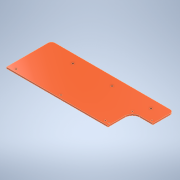
# Autodesk Inventor part: Electronics cover
Saved by Autodesk Inventor 2021 (Build 250183000, 183)
## iProperties
Created: 2020-08-17
Part Number: Electronics cover
Material: Generic
Document SubType Name: Modeling
Designer: jgray
Density: 1 g/cm^3
Appearance: Smooth - Light Orange
Author: jgray
Autodesk Inventor part; units mm, degrees
ref_plane "YZ Plane" through (0, 0, 0) normal (1, 0, 0) x (0, 1, 0)
ref_plane "XZ Plane" through (0, 0, 0) normal (0, 1, 0) x (-1, 0, 0)
ref_plane "XY Plane" through (0, 0, 0) normal (0, 0, 1) x (1, 0, 0)
sketch "Sketch1" plane through (0, 0, 0) normal (0, 1, 0) x (-1, 0, 0)
  line L0 (0, 0) -> (250, 0)
  line L1 (250, 0) -> (250, -85.25)
  line L2 (243, -92.25) -> (7, -92.25)
  line L3 (0, -85.25) -> (0, 0)
  arc A0 (243, -92.25) -> (250, -85.25) centre (243, -85.25) ccw
  arc A1 (0, -85.25) -> (7, -92.25) centre (7, -85.25) ccw
  point P0 (250, -92.25)
  point P1 (0, -92.25)
  dimension "d0" = 250
  dimension "d1" = 92.25
  dimension "d2" = 7
  constraints: 8 end point, 4 point on circle, 4 point on line, 4 tangent, 2 centre point, 2 parallel, 1 equal radius, 1 horizontal, 1 perpendicular
  measures "d0" distance of point (250, -92.25) point (0, -92.25)
  measures "d1" distance of L0.end point (250, -92.25)
  measures "d2" radius of A0
extrude "Extrusion1" add sketch "Sketch1" along normal blind 3
sketch "Sketch2" plane through (0, 3, 0) normal (0, 1, 0) x (1, 0, 0)
  line L0 (-302.172, 6) -> (59.9962, 6) construction
  line L1 (-309.1368, 74) -> (37.3606, 74) construction
  line L2 (-7, 92.25) -> (-243, 92.25) projected
  line L3 (-250, 0) -> (0, 0) projected
  line L4 (0, 0) -> (0, 85.25) projected
  line L5 (-250, 85.25) -> (-250, 0) projected
  point P0 (-28, 74)
  point P1 (-108, 74)
  point P2 (-188, 74)
  point P3 (-53.5, 6)
  point P4 (-144.5, 6)
  point P5 (-236.5, 6)
  dimension "d5" = 18.25
  dimension "d6" = 6
  dimension "d8" = 80
  dimension "d9" = 80
  dimension "d20" = 13.5
  dimension "d22" = 196.5
  dimension "d23" = 62
  dimension "d24" = 105.5
  constraints: 6 point on line, 4 end point, 2 horizontal
  measures "d5" distance between parallel lines of L2 L1
  measures "d6" distance between parallel lines of L3 L0
  measures "d8" distance of point (-28, 74) point (-108, 74)
  measures "d9" distance of point (-108, 74) point (-188, 74)
  measures "d20" distance from line of L5 point (-236.5, 6)
  measures "d22" distance from line of L5 point (-53.5, 6)
  measures "d23" distance from line of L5 point (-188, 74)
  measures "d24" distance from line of L5 point (-144.5, 6)
hole "Hole1" at (-28, 3, -74) at (-108, 3, -74) at (-188, 3, -74) at (-53.5, 3, -6) at (-144.5, 3, -6) at (-236.5, 3, -6) direction (0, -1, 0) diameter 3.8 end through all
sketch "Sketch3" plane through (0, 3, 0) normal (0, 1, 0) x (1, 0, 0)
  line L0 (0, 0) -> (-42, 0)
  line L1 (-42, 0) -> (-42, 35)
  line L2 (-27, 50) -> (0, 50)
  line L3 (0, 50) -> (0, 0)
  line L4 (-250, 85.25) -> (-250, 0) projected
  arc A0 (-27, 50) -> (-42, 35) centre (-27, 35) ccw
  dimension "d26" = 50
  dimension "d27" = 208
  dimension "d28" = 15
  constraints: 8 end point, 2 parallel, 2 point on circle, 2 tangent, 1 centre point, 1 horizontal, 1 perpendicular
  measures "d26" distance between parallel lines of L0 L2
  measures "d27" distance between parallel lines of L4 L1
  measures "d28" radius of A0
extrude "Extrusion2" cut sketch "Sketch3" against normal through all
sketch "Sketch4" plane through (0, 3, 0) normal (0, 1, 0) x (1, 0, 0)
  line L0 (-46, -14.9041) -> (-46, 62.5179) construction
  line L1 (7.7091, 54) -> (-71.6012, 54) construction
  line L2 (0, 50) -> (-27, 50) construction
  line L3 (0, 50) -> (-74.4337, 50) construction
  line L4 (-250, 0) -> (-42, 0) construction
  line L5 (-42, 0) -> (-42, 52.8873) construction
  line L6 (0, 50) -> (0, 85.25) projected
  point P0 (0, 0)
  point P1 (-6, 54)
  point P2 (-18, 54)
  point P3 (-46, 18)
  point P4 (-46, 6)
  point P5 (-42, 50)
  dimension "d31" = 4
  dimension "d32" = 4
  dimension "d33" = 6
  dimension "d34" = 6
  dimension "d35" = 18
  dimension "d36" = 18
  constraints: 8 end point, 6 point on line, 2 horizontal, 1 perpendicular, 1 vertical
  measures "d31" distance between parallel lines of L2 L1
  measures "d32" distance between parallel lines of L5 L0
  measures "d33" distance from line of L6 point (-6, 54)
  measures "d34" vertical distance of L4.end point (-46, 6)
  measures "d35" vertical distance of L4.end point (-46, 18)
  measures "d36" horizontal distance of L2.start point (-18, 54)
hole "Hole2" at (-6, 3, -54) at (-46, 3, -6) at (-42, 3, -50) direction (0, -1, 0) diameter 3.2 end through all
body "Solid1"
